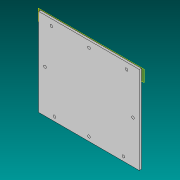
# Autodesk Inventor part: UP
Saved by Autodesk Inventor 2019 (Build 230136000, 136)
## iProperties
Created: 2025-01-01
Part Number: UP
Material: Generic
Document SubType Name: Modeling
Designer: Familia CS
Density: 1 g/cm^3
Appearance: Default
Author: Familia CS
Autodesk Inventor part; units mm, degrees
ref_plane "YZ Plane" through (0, 0, 0) normal (1, 0, 0) x (0, 1, 0)
ref_plane "XZ Plane" through (0, 0, 0) normal (0, 1, 0) x (-1, 0, 0)
ref_plane "XY Plane" through (0, 0, 0) normal (0, 0, 1) x (1, 0, 0)
ref_plane "Work Plane1" through (0, 0, 0) normal (0, 0, 1) x (1, 0, 0)
sketch "Sketch1" plane through (0, 0, 0) normal (0, 0, 1) x (1, 0, 0)
  line L0 (93, -80.5) -> (83, -80.5) projected
  line L1 (93, 2) -> (93, -80.5) projected
  line L2 (-2, -80.5) -> (-2, 2) projected
  line L3 (0, 2) -> (-2, 2) projected
  circle A0 centre (45.5, -4) radius 0.75 projected
  circle A1 centre (81, -4) radius 0.75 projected
  circle A2 centre (10, -4) radius 0.75 projected
  circle A3 centre (4, -40.25) radius 0.75 projected
  circle A4 centre (4, -70.5) radius 0.75 projected
  circle A5 centre (87, -40.25) radius 0.75 projected
  circle A6 centre (81, -76.5) radius 1.25 projected
  circle A7 centre (45.5, -76.5) radius 1.25 projected
  circle A8 centre (10, -76.5) radius 1.25 projected
  line L4 (93, -80.5) -> (-2, -80.5)
  line L5 (-2, -80.5) -> (-2, 2)
  line L6 (-2, 2) -> (93, 2)
  line L7 (93, 2) -> (93, -80.5)
  point P0 (0, 0)
  point P1 (87.75, -75.5)
  constraints: 8 end point, 2 parallel, 1 horizontal, 1 perpendicular, 1 other
extrude "Extrusion1" add sketch "Sketch1" along normal blind 2
sketch "Sketch2" plane through (0, 0, 2) normal (0, 0, 1) x (1, 0, 0)
  circle A0 centre (4, -70.5) radius 0.75 projected
  circle A1 centre (4, -70.5) radius 1.25
  circle A2 centre (4, -40.25) radius 0.75 projected
  circle A3 centre (4, -40.25) radius 1.25
  circle A4 centre (10, -4) radius 0.75 projected
  circle A5 centre (10, -4) radius 1.25
  circle A6 centre (45.5, -4) radius 0.75 projected
  circle A7 centre (45.5, -4) radius 1.25
  circle A8 centre (81, -4) radius 0.75 projected
  circle A9 centre (81, -4) radius 1.25
  circle A10 centre (87, -40.25) radius 0.75 projected
  circle A11 centre (87, -40.25) radius 1.25
  point P0 (0, 0)
  dimension "d2" = 2.5
  dimension "d3" = 2.5
  dimension "d4" = 2.5
  dimension "d5" = 2.5
  dimension "d6" = 2.5
  dimension "d7" = 2.5
  constraints: 6 centre point, 6 coincident
  measures "d2" diameter of A1
  measures "d3" diameter of A3
  measures "d4" diameter of A5
  measures "d5" diameter of A7
  measures "d6" diameter of A9
  measures "d7" diameter of A11
extrude "Extrusion2" cut sketch "Sketch2" against normal blind 2
sketch "Sketch3" plane through (0, 0, 2) normal (0, 0, 1) x (1, 0, 0)
  circle A0 centre (4, -70.5) radius 1.25 projected
  circle A1 centre (4, -70.5) radius 1.25
  point P0 (0, 0)
  constraints: 1 centre point, 1 coincident
extrude "Extrusion3" add sketch "Sketch3" against normal blind 2
sketch "Sketch4" plane through (0, 0, 2) normal (0, 0, 1) x (1, 0, 0)
  line L0 (8.2244, -73.6994) -> (84.6233, -73.6994)
  line L1 (84.6233, -73.6994) -> (84.6233, -78.8307)
  line L2 (84.6233, -78.8307) -> (8.2244, -78.8307)
  line L3 (8.2244, -78.8307) -> (8.2244, -73.6994)
  point P0 (0, 0)
  constraints: 8 end point, 2 parallel, 1 horizontal, 1 perpendicular
extrude "Extrusion4" add sketch "Sketch4" against normal blind 2
sketch "Sketch5" plane through (0, 0, 2) normal (0, 0, 1) x (1, 0, 0)
  line L0 (3.25, -80.5) -> (3.25, -75.5)
  line L1 (83, -80.5) -> (83, -65.5) projected
  circle A0 centre (45.5, -76.5) radius 1.25 projected
  line L2 (83, -72.5) -> (83, -80.5)
  circle A1 centre (78, -76.5) radius 1.25
  line L3 (8, -80.5) -> (8, -65.5) projected
  line L4 (8, -72.5) -> (8, -80.5)
  circle A2 centre (13, -76.5) radius 1.25
  point P0 (0, 0)
  dimension "d21" = 2.5
  dimension "d25" = 2.5
  constraints: 6 end point, 2 centre point, 1 vertical, 2 other
  measures "d21" diameter of A1
  measures "d25" diameter of A2
extrude "Extrusion5" cut sketch "Sketch5" against normal blind 2
body "Solid1"
